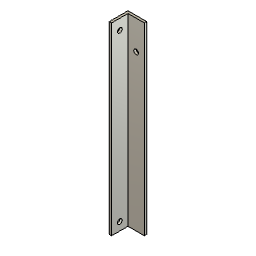
Angle 250 mm 1st Standing v13 (Autodesk Fusion 360 design; units mm, degrees)
Autodesk Fusion 360 part; units mm, degrees
sketch "Sketch1" plane through (0, 0, 0) normal (0, 1, 0) x (1, 0, 0)
  line L0 (0, -25.4) -> (0, 0)
  line L1 (0, 0) -> (25.4, 0)
  line L2 (12.7, -12.7) -> (11.05, -11.05) construction
  line L3 (3.175, -25.4) -> (3.175, -3.175)
  line L4 (3.175, -3.175) -> (25.4, -3.175)
  line L5 (25.4, -3.175) -> (25.4, 0)
  line L6 (0, -25.4) -> (3.175, -25.4)
  dimension "d1" = 25.4
  dimension "d2" = 25.4
  dimension "d13" = 3.175
  constraint coincident L0.end L2
  constraint coincident L0.end L1.start
  constraint perpendicular L1 L5
  constraint perpendicular L0 L1
  constraint vertical L0
  measures "d1" distance of L0.end L1.end
  measures "d2" distance of L0.start L0.end
extrude "Extrude1" add sketch "Sketch1" along normal blind 250
sketch "Sketch2" plane through (3.175, 0, 0) normal (1, 0, 0) x (0, 0, -1)
  line L0 (-25.4, 0) -> (-3.175, 0)
  line L1 (-3.175, 0) -> (-3.175, 250)
  line L2 (-3.175, 250) -> (-25.4, 250)
  line L3 (-25.4, 250) -> (-25.4, 0)
  circle A0 centre (-14.2875, 235.712) radius 2.76
  circle A1 centre (-14.2875, 11.1125) radius 2.5546
  line L4 (-14.2875, 250) -> (-14.2875, 0) construction
  dimension "d14" = 14.288
  dimension "d15" = 11.1125
  constraint vertical A0.centre A1.centre
  constraint midpoint L2 L4.start
  constraint midpoint L0 L4.end
  constraint coincident A1.centre L4
  measures "d14" distance of L2 A0.centre
  measures "d15" distance of L0 A1.centre
hole "Hole1" at (3.175, 11.1125, 14.2875) at (3.175, 235.712, 14.2875) direction (-1, 0, 0) diameter 6.5 end through all
hole "Hole2" at (14.287, 210.312, 3.175) direction (0, 0, -1) diameter 6.5 end through all
equation "d15 = ( 22.225 / 2 ) * 1 mm"
